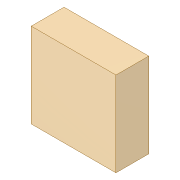
# Autodesk Inventor part: aerogelHolder
Saved by Autodesk Inventor 2017 (Build 210142000, 142)
## iProperties
Created: 2016-06-05
Part Number: aerogelHolder
Material: Polyethylene, Low Density
Document SubType Name: Modeling
Designer: sawaiz
Density: 0.894 g/cm^3
Appearance: Smooth - Off-White
Author: sawaiz
Autodesk Inventor part; units mm, degrees
ref_plane "YZ Plane" through (0, 0, 0) normal (1, 0, 0) x (0, 1, 0)
ref_plane "XZ Plane" through (0, 0, 0) normal (0, 1, 0) x (-1, 0, 0)
ref_plane "XY Plane" through (0, 0, 0) normal (0, 0, 1) x (1, 0, 0)
sketch "Sketch1" plane through (0, 0, 0) normal (0, 0, 1) x (1, 0, 0)
  line L0 (-63.5, -63.5) -> (63.5, -63.5)
  line L1 (63.5, -63.5) -> (63.5, 63.5)
  line L2 (63.5, 63.5) -> (-63.5, 63.5)
  line L3 (-63.5, 63.5) -> (-63.5, -63.5)
  line L4 (-63.5, -63.5) -> (63.5, 63.5) construction
  line L5 (63.5, -63.5) -> (-63.5, 63.5) construction
  point P0 (0, 0)
  dimension "d0" = 127
  dimension "d1" = 127
  constraints: 12 end point, 2 midpoint, 2 parallel, 1 horizontal, 1 perpendicular
  measures "d0" distance of L2.end L1.end
  measures "d1" distance of L1.end L0.end
extrude "Extrusion1" add sketch "Sketch1" along normal blind 49.2125
sketch "Sketch2" plane through (0, 0, 0) normal (0, 0, -1) x (-1, 0, 0)
  line L0 (-55, -55) -> (55, -55)
  line L1 (55, -55) -> (55, 55)
  line L2 (55, 55) -> (-55, 55)
  line L3 (-55, 55) -> (-55, -55)
  line L4 (-55, -55) -> (55, 55) construction
  line L5 (55, -55) -> (-55, 55) construction
  point P0 (0, 0)
  dimension "d4" = 110
  dimension "d5" = 110
  constraints: 12 end point, 2 midpoint, 2 parallel, 1 horizontal, 1 perpendicular
  measures "d4" distance of L2.end L1.end
  measures "d5" distance of L1.end L0.end
extrude "Extrusion2" cut sketch "Sketch2" against normal blind 30
equation "\"d0\" = width"
equation "\"d1\" = height"
equation "\"d2\" = aerogelHolderDepth"
equation "\"d4\" = aerogelWidth"
equation "\"d5\" = aerogelHeight"
equation "\"d6\" = aerogelThickness"
equation "\"plasticThickness\" = 6.35"
equation "\"aerogelThickness\" = 30"
equation "\"aerogelWidth\" = 110"
equation "\"aerogelHeight\" = 110"
equation "\"aerogelHolderDepth\" = 49.2125"
equation "\"height\" = 127"
equation "\"width\" = 127"
equation "\"depth\" = 203.2"
equation "\"mirrorAngle\" = 2.5deg"
equation "\"mirrorThickness\" = 3.175"
equation "\"fresnelThickness\" = 0.254"
equation "\"focalLength\" = 152.4"
equation "\"ior\" = 1.49"
equation "\"centerThickness\" = 1.27"
equation "\"fresnelAngle\" = 90deg"
equation "\"fresnelEffectiveDiameter\" = 152.4"
equation "\"caseThickness\" = 6.35"
equation "\"alignmentGrooveDepth\" = 1.5875"
equation "\"alignmentGrooveClearance\" = 0.1016"
equation "\"frontPanelThickness\" = 1.5875"
body "Solid1"
